Autodesk Fusion 360 part; units mm, degrees
(part 13 of 25)
  line L970 (11.6574, 39.243) -> (5.5534, 39.243)
  arc A2948 (37.4455, 40.2654) -> (37.4455, 40.5829) centre (37.4455, 40.4241) ccw
  line L971 (12.0775, 39.069) -> (11.6574, 39.243)
  line L972 (15.3804, 34.8514) -> (15.113, 35.1188)
  arc A2949 (35.1854, 41.2945) -> (35.5029, 41.2945) centre (35.3441, 41.2945) ccw
  line L973 (15.6337, 33.5781) -> (15.6337, 34.2399)
  line L974 (27.2855, 40.4241) -> (28.1559, 41.2945)
  arc A2950 (38.4746, 42.5255) -> (38.1571, 42.5255) centre (38.3158, 42.5255) ccw
  arc A2951 (5.4412, 39.1307) -> (5.6657, 39.3553) centre (5.5535, 39.243) ccw
  line L975 (26.5671, 40.4241) -> (27.2855, 40.4241)
  line L976 (35.3441, 41.2945) -> (36.2145, 40.4241)
  arc A2952 (14.9663, 35.7266) -> (15.2597, 35.8481) centre (15.113, 35.7874) ccw
  line L977 (36.2145, 40.4241) -> (37.4455, 40.4241)
  arc A2953 (12.1897, 39.1812) -> (11.9652, 38.9567) centre (12.0775, 39.069) ccw
  arc A2954 (38.2036, 42.4132) -> (38.4282, 42.6377) centre (38.3159, 42.5255) ccw
  arc A2955 (12.0167, 38.9223) -> (12.1382, 39.2157) centre (12.0775, 39.069) ccw
  arc A2956 (26.5671, 40.5829) -> (26.5671, 40.2654) centre (26.5671, 40.4241) ccw
  arc A2957 (36.3268, 43.2836) -> (36.1023, 43.5082) centre (36.2145, 43.3959) ccw
  arc A2958 (36.2145, 40.5829) -> (36.2145, 40.2654) centre (36.2145, 40.4241) ccw
  arc A2959 (15.2253, 35.2311) -> (15.0007, 35.0066) centre (15.113, 35.1189) ccw
  line L978 (15.6337, 34.2399) -> (15.3804, 34.8514)
  arc A2960 (15.2682, 34.7392) -> (15.4927, 34.9637) centre (15.3805, 34.8514) ccw
  arc A2961 (37.5577, 43.5082) -> (37.3332, 43.2836) centre (37.4455, 43.3959) ccw
  arc A2962 (4.8214, 43.6691) -> (5.1147, 43.5476) centre (4.968, 43.6084) ccw
  arc A2963 (14.9542, 35.1188) -> (15.2717, 35.1188) centre (15.113, 35.1188) ccw
  line L979 (5.1943, 44.7456) -> (4.9681, 45.2917)
  line L980 (0.9017, 44.1544) -> (1.1279, 43.6083)
  arc A2964 (4.4378, 43.3026) -> (4.6623, 43.0781) centre (4.55, 43.1903) ccw
  arc A2965 (0.9812, 43.5476) -> (1.2746, 43.6691) centre (1.1279, 43.6084) ccw
  line L981 (5.1943, 42.2056) -> (4.9681, 42.7517)
  arc A2966 (1.0157, 45.4039) -> (1.2402, 45.1794) centre (1.128, 45.2917) ccw
  arc A2967 (0.755, 44.8063) -> (1.0484, 44.6848) centre (0.9017, 44.7456) ccw
  arc A2968 (4.2037, 40.6787) -> (4.3252, 40.3853) centre (4.2645, 40.532) ccw
  arc A2969 (5.341, 41.5537) -> (5.0476, 41.6752) centre (5.1943, 41.6145) ccw
  line L982 (4.9681, 42.7517) -> (4.5501, 43.1697)
  line L983 (1.5459, 45.7097) -> (1.1279, 45.2917)
  line L984 (1.5459, 43.1903) -> (1.5708, 43.18)
  arc A2970 (1.6582, 45.5974) -> (1.4336, 45.8219) centre (1.5459, 45.7097) ccw
  arc A2971 (4.0647, 46.0826) -> (3.9432, 45.7892) centre (4.004, 45.9359) ccw
  line L985 (4.9681, 45.2917) -> (4.5501, 45.7097)
  arc A2972 (1.2402, 43.7206) -> (1.0157, 43.496) centre (1.1279, 43.6083) ccw
  arc A2973 (0.7429, 44.1544) -> (1.0605, 44.1544) centre (0.9017, 44.1544) ccw
  arc A2974 (5.0803, 40.956) -> (4.8558, 41.1806) centre (4.9681, 41.0683) ccw
  line L986 (4.5501, 43.1903) -> (4.9681, 43.6083)
  line L987 (1.1279, 43.6083) -> (1.5459, 43.1903)
  line L988 (5.1943, 41.6144) -> (5.1943, 42.2056)
  arc A2975 (5.0355, 41.6144) -> (5.353, 41.6144) centre (5.1943, 41.6144) ccw
  arc A2976 (4.6108, 43.0436) -> (4.4894, 43.337) centre (4.5501, 43.1903) ccw
  line L989 (2.092, 45.9359) -> (1.5459, 45.7097)
  arc A2977 (5.341, 44.0937) -> (5.0476, 44.2152) centre (5.1943, 44.1544) ccw
  arc A2978 (4.4893, 45.563) -> (4.6108, 45.8563) centre (4.5501, 45.7097) ccw
  line L990 (4.5501, 43.1697) -> (4.5252, 43.18)
  arc A2979 (2.092, 46.0946) -> (2.092, 45.7771) centre (2.092, 45.9359) ccw
  line L991 (0.9017, 44.7456) -> (0.9017, 44.1544)
  line L992 (1.1279, 45.2917) -> (0.9017, 44.7456)
  arc A2980 (5.0355, 44.1544) -> (5.353, 44.1544) centre (5.1943, 44.1544) ccw
  arc A2981 (4.8558, 45.1794) -> (5.0803, 45.4039) centre (4.9681, 45.2917) ccw
  arc A2982 (4.4644, 43.3267) -> (4.5859, 43.0333) centre (4.5251, 43.18) ccw
  arc A2983 (1.4336, 43.0781) -> (1.6582, 43.3026) centre (1.5459, 43.1904) ccw
  arc A2984 (4.4893, 43.023) -> (4.6108, 43.3163) centre (4.55, 43.1696) ccw
  arc A2985 (1.0605, 44.7456) -> (0.7429, 44.7456) centre (0.9017, 44.7456) ccw
  line L993 (4.5501, 45.7097) -> (4.004, 45.9359)
  arc A2986 (5.353, 42.2056) -> (5.0355, 42.2056) centre (5.1943, 42.2056) ccw
  arc A2987 (1.0484, 44.2152) -> (0.755, 44.0937) centre (0.9017, 44.1544) ccw
  line L994 (4.9681, 41.0683) -> (5.1943, 41.6144)
  arc A2988 (5.1147, 42.8124) -> (4.8214, 42.6909) centre (4.9681, 42.7516) ccw
  arc A2989 (4.8558, 42.6394) -> (5.0803, 42.8639) centre (4.968, 42.7517) ccw
  line L995 (4.5252, 43.18) -> (4.5501, 43.1903)
  arc A2990 (5.0476, 44.6848) -> (5.341, 44.8063) centre (5.1943, 44.7456) ccw
  arc A2991 (4.5859, 43.3267) -> (4.4644, 43.0333) centre (4.5251, 43.18) ccw
  arc A2992 (5.1147, 45.3524) -> (4.8214, 45.2309) centre (4.968, 45.2916) ccw
  arc A2993 (2.1528, 45.7892) -> (2.0313, 46.0826) centre (2.0921, 45.9359) ccw
  arc A2994 (5.353, 44.7456) -> (5.0355, 44.7456) centre (5.1943, 44.7456) ccw
  arc A2995 (4.6108, 40.5036) -> (4.4893, 40.797) centre (4.5501, 40.6503) ccw
  arc A2996 (4.6623, 45.8219) -> (4.4378, 45.5974) centre (4.5501, 45.7097) ccw
  arc A2997 (5.0803, 43.496) -> (4.8558, 43.7206) centre (4.968, 43.6083) ccw
  arc A2998 (5.0476, 42.1448) -> (5.341, 42.2663) centre (5.1943, 42.2056) ccw
  line L996 (5.1943, 44.1544) -> (5.1943, 44.7456)
  arc A2999 (4.8214, 41.1291) -> (5.1147, 41.0076) centre (4.9681, 41.0684) ccw
  line L997 (4.2644, 40.532) -> (4.5501, 40.6503)
  line L998 (4.5501, 40.6503) -> (4.9681, 41.0683)
  arc A3000 (4.004, 45.7771) -> (4.004, 46.0946) centre (4.004, 45.9359) ccw
  arc A3001 (4.6623, 43.2819) -> (4.4378, 43.0574) centre (4.55, 43.1696) ccw
  arc A3002 (1.4852, 45.8563) -> (1.6067, 45.563) centre (1.5459, 45.7097) ccw
  arc A3003 (1.2746, 45.2309) -> (0.9812, 45.3524) centre (1.1279, 45.2917) ccw
  line L999 (4.004, 45.9359) -> (2.092, 45.9359)
  line L1000 (4.9681, 43.6083) -> (5.1943, 44.1544)
  line L1001 (0.9017, 41.6144) -> (1.1279, 41.0683)
  arc A3004 (1.0605, 42.2056) -> (0.7429, 42.2056) centre (0.9017, 42.2056) ccw
  line L1002 (10.9566, 36.957) -> (12.8109, 35.1027)
  arc A3005 (1.9323, 39.4238) -> (2.2257, 39.5453) centre (2.079, 39.4845) ccw
  line L1003 (1.1279, 41.0683) -> (1.5459, 40.6503)
  arc A3006 (1.4851, 43.3163) -> (1.6067, 43.023) centre (1.5459, 43.1696) ccw
  arc A3007 (2.0638, 40.5016) -> (1.7463, 40.5016) centre (1.9051, 40.5016) ccw
  line L1004 (12.8109, 35.1027) -> (12.5596, 34.8514)
  arc A3008 (0.755, 42.2663) -> (1.0484, 42.1448) centre (0.9017, 42.2056) ccw
  arc A3009 (12.4473, 34.9637) -> (12.6718, 34.7392) centre (12.5595, 34.8514) ccw
  arc A3010 (1.6066, 43.337) -> (1.4852, 43.0436) centre (1.5459, 43.1903) ccw
  arc A3011 (4.2233, 37.5648) -> (3.9988, 37.3403) centre (4.111, 37.4526) ccw
  arc A3012 (1.6316, 43.0333) -> (1.5101, 43.3267) centre (1.5708, 43.18) ccw
  arc A3013 (1.6582, 43.0574) -> (1.4336, 43.2819) centre (1.5459, 43.1696) ccw
  line L1005 (4.111, 37.4525) -> (4.4325, 37.131)
  line L1006 (1.905, 39.9046) -> (2.079, 39.4845)
  arc A3014 (1.5101, 43.0333) -> (1.6316, 43.3267) centre (1.5709, 43.18) ccw
  arc A3015 (12.465, 34.2399) -> (12.1476, 34.2399) centre (12.3063, 34.2399) ccw
  arc A3016 (4.7919, 36.8103) -> (4.9134, 37.1037) centre (4.8527, 36.957) ccw
  arc A3017 (4.3203, 37.0188) -> (4.5448, 37.2433) centre (4.4325, 37.1311) ccw
  arc A3018 (1.2402, 41.1806) -> (1.0157, 40.956) centre (1.128, 41.0683) ccw
  arc A3019 (4.4933, 37.2777) -> (4.3718, 36.9843) centre (4.4326, 37.131) ccw
  arc A3020 (1.0157, 42.8639) -> (1.2402, 42.6394) centre (1.128, 42.7517) ccw
  line L1007 (1.5708, 43.18) -> (1.5459, 43.1697)
  arc A3021 (1.0484, 41.6752) -> (0.755, 41.5537) centre (0.9017, 41.6145) ccw
  line L1008 (4.8526, 36.957) -> (10.9566, 36.957)
  line L1009 (1.905, 40.5016) -> (1.905, 39.9046)
  arc A3022 (11.0688, 37.0693) -> (10.8443, 36.8447) centre (10.9566, 36.957) ccw
  arc A3023 (4.4378, 40.7626) -> (4.6623, 40.5381) centre (4.55, 40.6504) ccw
  arc A3024 (1.8442, 40.3549) -> (1.9658, 40.6482) centre (1.905, 40.5016) ccw
  arc A3025 (1.2746, 42.6909) -> (0.9812, 42.8124) centre (1.1279, 42.7516) ccw
  arc A3026 (2.0517, 39.9654) -> (1.7583, 39.8439) centre (1.905, 39.9047) ccw
  arc A3027 (12.1596, 34.3007) -> (12.453, 34.1792) centre (12.3063, 34.24) ccw
  line L1010 (1.5459, 40.6503) -> (1.905, 40.5016)
  arc A3028 (1.4336, 40.5381) -> (1.6582, 40.7626) centre (1.5459, 40.6504) ccw
  arc A3029 (12.9231, 34.9904) -> (12.6986, 35.2149) centre (12.8109, 35.1027) ccw
  line L1011 (0.9017, 42.2056) -> (0.9017, 41.6144)
  line L1012 (12.5596, 34.8514) -> (12.3063, 34.2399)
  line L1013 (1.5459, 43.1697) -> (1.1279, 42.7517)
  line L1014 (2.079, 39.4845) -> (4.111, 37.4525)
  arc A3030 (4.8526, 37.1157) -> (4.8526, 36.7983) centre (4.8526, 36.957) ccw
  line L1015 (4.4325, 37.131) -> (4.8526, 36.957)
  arc A3031 (0.9812, 41.0076) -> (1.2746, 41.1291) centre (1.1279, 41.0684) ccw
  arc A3032 (0.7429, 41.6144) -> (1.0605, 41.6144) centre (0.9017, 41.6144) ccw
  arc A3033 (3.9988, 37.3403) -> (4.2233, 37.5648) centre (4.111, 37.4526) ccw
  arc A3034 (10.9566, 36.7983) -> (10.9566, 37.1157) centre (10.9566, 36.957) ccw
  arc A3035 (1.7463, 39.9046) -> (2.0638, 39.9046) centre (1.9051, 39.9046) ccw
  arc A3036 (1.6067, 40.797) -> (1.4852, 40.5036) centre (1.5459, 40.6503) ccw
  line L1016 (1.1279, 42.7517) -> (0.9017, 42.2056)
  arc A3037 (15.2337, 33.0273) -> (15.5271, 32.9058) centre (15.3804, 32.9666) ccw
  line L1017 (15.3797, 3.81) -> (15.3797, 4.3939)
  arc A3038 (15.7459, 5.5486) -> (15.5214, 5.7731) centre (15.6337, 5.6609) ccw
  arc A3039 (13.8112, 2.4003) -> (14.1287, 2.4003) centre (13.97, 2.4003) ccw
  arc A3040 (12.6986, 34.9904) -> (12.9231, 35.2149) centre (12.8109, 35.1027) ccw
  line L1018 (15.3804, 32.9666) -> (15.6337, 33.5781)
  arc A3041 (13.0883, 32.6452) -> (12.9668, 32.3519) centre (13.0275, 32.4986) ccw
  arc A3042 (13.97, 3.9688) -> (13.97, 3.6513) centre (13.97, 3.81) ccw
  arc A3043 (13.97, 3.9687) -> (13.97, 3.6512) centre (13.97, 3.81) ccw
  line L1019 (14.5539, 2.4003) -> (15.3797, 3.2261)
  arc A3044 (15.3797, 3.6513) -> (15.3797, 3.9688) centre (15.3797, 3.81) ccw
  arc A3045 (15.7804, 33.5173) -> (15.487, 33.6388) centre (15.6337, 33.578) ccw
  arc A3046 (13.6391, 32.404) -> (13.6391, 32.0866) centre (13.6391, 32.2453) ccw
  line L1020 (13.97, 2.4003) -> (13.97, 3.81)
  arc A3047 (12.6718, 33.0788) -> (12.4473, 32.8543) centre (12.5596, 32.9666) ccw
  arc A3048 (15.2209, 3.81) -> (15.5384, 3.81) centre (15.3796, 3.81) ccw
  line L1021 (13.0276, 32.4986) -> (13.6391, 32.2453)
  line L1022 (15.3797, 4.3939) -> (14.8732, 4.9004)
  arc A3049 (15.2674, 4.2817) -> (15.492, 4.5062) centre (15.3797, 4.394) ccw
  arc A3050 (13.97, 3.9687) -> (13.97, 3.6512) centre (13.97, 3.81) ccw
  arc A3051 (15.5384, 4.3939) -> (15.2209, 4.3939) centre (15.3796, 4.3939) ccw
  arc A3052 (2.1913, 39.5968) -> (1.9668, 39.3723) centre (2.0791, 39.4846) ccw
  line L1023 (13.97, 3.81) -> (15.3797, 3.81)
  line L1024 (14.8732, 4.9004) -> (15.6337, 5.6609)
  arc A3053 (14.9732, 32.3519) -> (14.8517, 32.6452) centre (14.9124, 32.4986) ccw
  arc A3054 (12.4129, 32.9058) -> (12.7062, 33.0273) centre (12.5596, 32.9666) ccw
  line L1025 (15.6337, 5.6609) -> (15.6337, 7.0391)
  arc A3055 (13.97, 2.2415) -> (13.97, 2.559) centre (13.97, 2.4003) ccw
  arc A3056 (15.5384, 3.81) -> (15.2209, 3.81) centre (15.3796, 3.81) ccw
  arc A3057 (12.453, 33.6388) -> (12.1596, 33.5173) centre (12.3063, 33.578) ccw
  line L1026 (12.5596, 32.9666) -> (13.0276, 32.4986)
  arc A3058 (13.97, 3.6512) -> (13.97, 3.9687) centre (13.97, 3.81) ccw
  arc A3059 (12.9153, 32.3863) -> (13.1398, 32.6108) centre (13.0275, 32.4986) ccw
  line L1027 (15.3797, 3.2261) -> (15.3797, 3.81)
  line L1028 (13.3861, 2.4003) -> (13.97, 2.4003)
  arc A3060 (10.7132, 8.4483) -> (10.4887, 8.2238) centre (10.601, 8.3361) ccw
  line L1029 (6.2035, 16.2179) -> (5.6955, 16.7259)
  arc A3061 (10.5988, 8.7562) -> (10.3054, 8.6347) centre (10.4521, 8.6955) ccw
  line L1030 (12.3063, 6.6307) -> (12.3063, 5.6609)
  arc A3062 (11.8717, 12.1468) -> (12.0962, 12.3713) centre (11.984, 12.2591) ccw
  arc A3063 (14.1288, 3.81) -> (13.8113, 3.81) centre (13.9701, 3.81) ccw
  line L1031 (14.3009, 32.2453) -> (14.9124, 32.4986)
  arc A3064 (15.2209, 3.2261) -> (15.5384, 3.2261) centre (15.3796, 3.2261) ccw
  line L1032 (4.4645, 13.7541) -> (5.6955, 13.7541)
  line L1033 (12.4079, 9.2951) -> (12.4079, 11.6245)
  arc A3065 (14.8002, 32.6108) -> (15.0247, 32.3863) centre (14.9125, 32.4986) ccw
  line L1034 (7.2149, 14.2621) -> (10.4521, 11.0249)
  arc A3066 (13.97, 2.5591) -> (13.97, 2.2416) centre (13.97, 2.4004) ccw
  arc A3067 (14.761, 5.0126) -> (14.9855, 4.7881) centre (14.8733, 4.9003) ccw
  arc A3068 (14.2402, 32.392) -> (14.3617, 32.0986) centre (14.301, 32.2453) ccw
  line L1035 (13.97, 3.81) -> (13.97, 2.4003)
  arc A3069 (13.3861, 2.559) -> (13.3861, 2.2416) centre (13.3861, 2.4003) ccw
  line L1036 (15.3797, 3.81) -> (13.97, 3.81)
  arc A3070 (13.5783, 32.0986) -> (13.6998, 32.392) centre (13.639, 32.2453) ccw
  arc A3071 (14.1288, 3.81) -> (13.8113, 3.81) centre (13.9701, 3.81) ccw
  arc A3072 (15.4927, 32.8543) -> (15.2682, 33.0788) centre (15.3804, 32.9666) ccw
  arc A3073 (4.4645, 13.9129) -> (4.4645, 13.5954) centre (4.4645, 13.7542) ccw
  arc A3074 (12.0962, 12.3713) -> (11.8717, 12.1468) centre (11.984, 12.2591) ccw
  arc A3075 (15.4749, 5.6609) -> (15.7924, 5.6609) centre (15.6337, 5.6609) ccw
  arc A3076 (8.2862, 16.1813) -> (8.0617, 15.9568) centre (8.1739, 16.0691) ccw
  arc A3077 (7.3272, 14.3744) -> (7.1027, 14.1498) centre (7.2149, 14.2621) ccw
  arc A3078 (15.492, 3.1138) -> (15.2674, 3.3383) centre (15.3797, 3.2261) ccw
  line L1037 (13.97, 2.4003) -> (14.5539, 2.4003)
  arc A3079 (14.9855, 5.0126) -> (14.761, 4.7881) centre (14.8733, 4.9003) ccw
  arc A3080 (14.1287, 3.81) -> (13.8112, 3.81) centre (13.97, 3.81) ccw
  line L1038 (14.9124, 32.4986) -> (15.3804, 32.9666)
  arc A3081 (7.8145, 16.0591) -> (7.8145, 16.3766) centre (7.8145, 16.2179) ccw
  arc A3082 (12.5666, 11.6245) -> (12.2491, 11.6245) centre (12.4078, 11.6245) ccw
  line L1039 (15.6337, 7.0391) -> (14.6591, 8.0137)
  line L1040 (12.4079, 11.6245) -> (12.259, 11.9839)
  arc A3083 (3.7529, 15.8555) -> (3.4354, 15.8555) centre (3.5941, 15.8555) ccw
  line L1041 (10.4521, 11.0249) -> (10.4521, 8.6955)
  arc A3084 (10.6108, 11.0249) -> (10.2934, 11.0249) centre (10.4521, 11.0249) ccw
  arc A3085 (10.4543, 8.2753) -> (10.7476, 8.3968) centre (10.601, 8.3361) ccw
  arc A3086 (72.6868, 22.0663) -> (72.6868, 22.3838) centre (72.6868, 22.2251) ccw
  arc A3087 (5.6955, 13.5954) -> (5.6955, 13.9129) centre (5.6955, 13.7542) ccw
  arc A3088 (14.3009, 32.0866) -> (14.3009, 32.404) centre (14.3009, 32.2453) ccw
  arc A3089 (56.8579, 22.3838) -> (56.8579, 22.0663) centre (56.8579, 22.2251) ccw
  arc A3090 (15.3797, 3.6512) -> (15.3797, 3.9687) centre (15.3797, 3.81) ccw
  arc A3091 (7.2149, 14.1034) -> (7.2149, 14.4208) centre (7.2149, 14.2621) ccw
  arc A3092 (14.5539, 2.2416) -> (14.5539, 2.5591) centre (14.5539, 2.4004) ccw
  arc A3093 (4.4645, 16.8846) -> (4.4645, 16.5671) centre (4.4645, 16.7259) ccw
  arc A3094 (15.7924, 7.0391) -> (15.4749, 7.0391) centre (15.6337, 7.0391) ccw
  arc A3095 (14.4417, 2.5126) -> (14.6662, 2.288) centre (14.554, 2.4003) ccw
  arc A3096 (13.8113, 3.81) -> (14.1288, 3.81) centre (13.9701, 3.81) ccw
  arc A3097 (13.8113, 2.4003) -> (14.1288, 2.4003) centre (13.9701, 2.4003) ccw
  line L1042 (13.6391, 32.2453) -> (14.3009, 32.2453)
  arc A3098 (6.2035, 16.3766) -> (6.2035, 16.0591) centre (6.2035, 16.2179) ccw
  line L1043 (3.5941, 14.6245) -> (4.4645, 13.7541)
  arc A3099 (12.1476, 5.6609) -> (12.465, 5.6609) centre (12.3063, 5.6609) ccw
  line L1044 (10.4521, 8.6955) -> (10.601, 8.3361)
  arc A3100 (44.8038, 14.6194) -> (44.5105, 14.7409) centre (44.6572, 14.6802) ccw
  arc A3101 (44.6251, 14.2194) -> (44.3076, 14.2194) centre (44.4664, 14.2194) ccw
  line L1045 (13.6893, 8.0137) -> (12.4079, 9.2951)
  line L1046 (12.5603, 3.2261) -> (13.3861, 2.4003)
  arc A3102 (12.2612, 11.5638) -> (12.5546, 11.6853) centre (12.4079, 11.6246) ccw
  line L1047 (13.0668, 4.9004) -> (12.5603, 4.3939)
  arc A3103 (45.5314, 15.077) -> (45.4099, 15.3704) centre (45.4706, 15.2237) ccw
  arc A3104 (3.4354, 14.6245) -> (3.7529, 14.6245) centre (3.5941, 14.6245) ccw
  line L1048 (44.4663, 13.7206) -> (44.6572, 13.2598)
  arc A3105 (13.6893, 8.1724) -> (13.6893, 7.8549) centre (13.6893, 8.0137) ccw
  arc A3106 (14.7714, 8.126) -> (14.5469, 7.9014) centre (14.6592, 8.0137) ccw
  arc A3107 (12.2491, 9.2951) -> (12.5666, 9.2951) centre (12.4078, 9.2951) ccw
  arc A3108 (6.2035, 14.4208) -> (6.2035, 14.1034) centre (6.2035, 14.2621) ccw
  line L1049 (3.5941, 15.8555) -> (3.5941, 14.6245)
  arc A3109 (8.1132, 15.9224) -> (8.2347, 16.2157) centre (8.1739, 16.0691) ccw
  arc A3110 (6.0912, 16.1056) -> (6.3157, 16.3302) centre (6.2035, 16.2179) ccw
  line L1050 (7.8145, 16.2179) -> (6.2035, 16.2179)
  arc A3111 (4.3523, 13.6418) -> (4.5768, 13.8664) centre (4.4646, 13.7541) ccw
  arc A3112 (12.5202, 9.4073) -> (12.2956, 9.1828) centre (12.4079, 9.2951) ccw
  arc A3113 (12.1468, 11.8717) -> (12.3713, 12.0962) centre (12.2591, 11.984) ccw
  arc A3114 (14.6591, 7.8549) -> (14.6591, 8.1724) centre (14.6591, 8.0137) ccw
  arc A3115 (7.8753, 16.3646) -> (7.7538, 16.0712) centre (7.8146, 16.2179) ccw
  arc A3116 (4.5768, 16.6136) -> (4.3523, 16.8382) centre (4.4645, 16.7259) ccw
  arc A3117 (10.3398, 10.9127) -> (10.5644, 11.1372) centre (10.4521, 11.025) ccw
  arc A3118 (5.6955, 16.5671) -> (5.6955, 16.8846) centre (5.6955, 16.7259) ccw
  line L1051 (14.6591, 8.0137) -> (13.6893, 8.0137)
  arc A3119 (5.5832, 13.8664) -> (5.8077, 13.6418) centre (5.6954, 13.7541) ccw
  arc A3120 (44.3076, 13.7206) -> (44.6251, 13.7206) centre (44.4664, 13.7206) ccw
  arc A3121 (44.3196, 14.2801) -> (44.613, 14.1586) centre (44.4663, 14.2193) ccw
  line L1052 (5.6955, 16.7259) -> (4.4645, 16.7259)
  arc A3122 (3.4818, 15.9677) -> (3.7064, 15.7432) centre (3.5941, 15.8554) ccw
  line L1053 (12.259, 11.9839) -> (11.9839, 12.259)
  arc A3123 (3.7064, 14.7368) -> (3.4818, 14.5123) centre (3.5941, 14.6246) ccw
  line L1054 (45.4706, 15.2237) -> (45.0098, 15.0328)
  arc A3124 (12.4057, 12.0447) -> (12.1124, 11.9232) centre (12.2591, 11.984) ccw
  arc A3125 (12.4016, 3.81) -> (12.719, 3.81) centre (12.5603, 3.81) ccw
  arc A3126 (14.1287, 3.81) -> (13.8112, 3.81) centre (13.97, 3.81) ccw
  line L1055 (12.5603, 3.81) -> (13.97, 3.81)
  line L1056 (5.6955, 13.7541) -> (6.2035, 14.2621)
  arc A3127 (5.8077, 16.8382) -> (5.5832, 16.6136) centre (5.6954, 16.7259) ccw
  line L1057 (12.3063, 5.6609) -> (13.0668, 4.9004)
  line L1058 (12.5603, 4.3939) -> (12.5603, 3.81)
  line L1059 (6.2035, 14.2621) -> (7.2149, 14.2621)
  line L1060 (8.1739, 16.069) -> (7.8145, 16.2179)
  arc A3128 (6.3157, 14.1498) -> (6.0912, 14.3744) centre (6.2035, 14.2621) ccw
  line L1061 (44.6572, 13.2598) -> (44.7421, 13.1749)
  line L1062 (10.601, 8.3361) -> (12.3063, 6.6307)
  arc A3129 (44.5105, 13.1991) -> (44.8038, 13.3206) centre (44.6572, 13.2599) ccw
  arc A3130 (10.2934, 8.6955) -> (10.6108, 8.6955) centre (10.4521, 8.6955) ccw
  line L1063 (11.9839, 12.259) -> (8.1739, 16.069)
  arc A3131 (12.4016, 3.2261) -> (12.719, 3.2261) centre (12.5603, 3.2261) ccw
  line L1064 (4.4645, 16.7259) -> (3.5941, 15.8555)
  arc A3132 (15.5214, 6.9269) -> (15.746, 7.1514) centre (15.6337, 7.0391) ccw
  arc A3133 (13.577, 7.9014) -> (13.8015, 8.1259) centre (13.6893, 8.0137) ccw
  arc A3134 (12.5603, 3.9688) -> (12.5603, 3.6513) centre (12.5603, 3.81) ccw
  arc A3135 (46.8149, 13.7206) -> (47.1324, 13.7206) centre (46.9737, 13.7206) ccw
  arc A3136 (12.194, 6.5185) -> (12.4186, 6.743) centre (12.3063, 6.6308) ccw
  arc A3137 (44.7694, 13.3721) -> (44.5449, 13.1476) centre (44.6571, 13.2599) ccw
  arc A3138 (12.465, 6.6307) -> (12.1476, 6.6307) centre (12.3063, 6.6307) ccw
  arc A3139 (44.6298, 13.0626) -> (44.8544, 13.2872) centre (44.7421, 13.1749) ccw
  line L1065 (44.7421, 13.1749) -> (44.7421, 7.8557)
  arc A3140 (44.8028, 7.709) -> (44.6814, 8.0024) centre (44.7421, 7.8557) ccw
  arc A3141 (44.9008, 13.1749) -> (44.5834, 13.1749) centre (44.7421, 13.1749) ccw
  arc A3142 (45.9694, 15.0649) -> (45.9694, 15.3824) centre (45.9694, 15.2236) ccw
  arc A3143 (13.2738, 2.288) -> (13.4983, 2.5126) centre (13.3861, 2.4003) ccw
  arc A3144 (40.0108, 7.9016) -> (40.1089, 7.5996) centre (40.0599, 7.7506) ccw
  arc A3145 (46.5424, 15.1451) -> (46.3179, 14.9206) centre (46.4301, 15.0329) ccw
  line L1066 (44.6572, 14.6802) -> (44.4663, 14.2194)
  arc A3146 (44.6593, 7.9932) -> (44.7808, 7.6999) centre (44.7201, 7.8466) ccw
  arc A3147 (43.5919, 8.262) -> (43.4704, 7.9686) centre (43.5312, 8.1153) ccw
  arc A3148 (44.1192, 7.6999) -> (44.2407, 7.9932) centre (44.1799, 7.8466) ccw
  arc A3149 (13.179, 4.7881) -> (12.9545, 5.0126) centre (13.0668, 4.9003) ccw
  arc A3150 (43.5311, 7.9565) -> (43.5311, 8.274) centre (43.5311, 8.1152) ccw
  arc A3151 (46.6706, 14.5679) -> (46.8951, 14.7924) centre (46.7829, 14.6801) ccw
  line L1067 (46.4302, 15.0328) -> (45.9694, 15.2237)
  arc A3152 (46.0301, 15.3704) -> (45.9086, 15.077) centre (45.9694, 15.2237) ccw
  line L1068 (45.9694, 15.2237) -> (45.4706, 15.2237)
  arc A3153 (46.9295, 14.7409) -> (46.6362, 14.6194) centre (46.7828, 14.6801) ccw
  arc A3154 (12.719, 4.3939) -> (12.4016, 4.3939) centre (12.5603, 4.3939) ccw
  line L1069 (12.5603, 3.81) -> (12.5603, 3.2261)
  arc A3155 (45.4706, 15.3824) -> (45.4706, 15.0649) centre (45.4706, 15.2236) ccw
  arc A3156 (47.1324, 14.2194) -> (46.8149, 14.2194) centre (46.9737, 14.2194) ccw
  arc A3157 (44.5834, 7.8557) -> (44.9008, 7.8557) centre (44.7421, 7.8557) ccw
  arc A3158 (12.6726, 3.3383) -> (12.448, 3.1138) centre (12.5603, 3.2261) ccw
  arc A3159 (13.97, 3.6513) -> (13.97, 3.9688) centre (13.97, 3.81) ccw
  line L1070 (46.9737, 14.2194) -> (46.7828, 14.6802)
  arc A3160 (46.3694, 14.8862) -> (46.4909, 15.1795) centre (46.4301, 15.0328) ccw
  arc A3161 (44.5449, 14.7924) -> (44.7694, 14.5679) centre (44.6571, 14.6802) ccw
  line L1071 (44.72, 7.8465) -> (44.45, 7.5765)
  line L1072 (44.7421, 7.8557) -> (44.72, 7.8465)
  line L1073 (44.4663, 14.2194) -> (44.4663, 13.7206)
  line L1074 (45.0098, 15.0328) -> (44.6572, 14.6802)
  line L1075 (39.6555, 7.5028) -> (39.4872, 7.3345)
  line L1076 (46.7828, 14.6802) -> (46.4302, 15.0328)
  arc A3162 (44.613, 13.7814) -> (44.3196, 13.6599) centre (44.4663, 13.7206) ccw
  arc A3163 (13.97, 3.6512) -> (13.97, 3.9687) centre (13.97, 3.81) ccw
  arc A3164 (12.4186, 5.7731) -> (12.194, 5.5486) centre (12.3063, 5.6609) ccw
  line L1077 (40.2861, 7.8241) -> (40.0599, 7.7506)
  line L1078 (46.9737, 13.7206) -> (46.9737, 14.2194)
  arc A3165 (41.6181, 7.5092) -> (41.8426, 7.2846) centre (41.7303, 7.3969) ccw
  arc A3166 (45.1221, 14.9206) -> (44.8976, 15.1451) centre (45.0099, 15.0328) ccw
  arc A3167 (39.375, 7.4468) -> (39.5995, 7.2223) centre (39.4873, 7.3346) ccw
  arc A3168 (12.719, 3.81) -> (12.4016, 3.81) centre (12.5603, 3.81) ccw
  arc A3169 (13.8112, 3.81) -> (14.1287, 3.81) centre (13.97, 3.81) ccw
  arc A3170 (40.9691, 7.6673) -> (41.0187, 7.9809) centre (40.9939, 7.8241) ccw
  line L1079 (43.5311, 8.1153) -> (42.8289, 8.1153)
  arc A3171 (42.8896, 7.9686) -> (42.7681, 8.262) centre (42.8289, 8.1153) ccw
  line L1080 (13.97, 3.81) -> (12.5603, 3.81)
  arc A3172 (44.9491, 15.1795) -> (45.0706, 14.8862) centre (45.0099, 15.0328) ccw
  arc A3173 (42.2923, 7.7343) -> (42.0678, 7.9588) centre (42.18, 7.8466) ccw
  arc A3174 (12.9545, 4.7881) -> (13.179, 5.0126) centre (13.0668, 4.9003) ccw
  arc A3175 (40.64, 8.02) -> (40.64, 7.7025) centre (40.64, 7.8613) ccw
  line L1081 (41.2201, 7.7506) -> (40.9939, 7.8241)
  arc A3176 (12.448, 4.5062) -> (12.6726, 4.2817) centre (12.5603, 4.394) ccw
  line L1082 (40.9939, 7.8241) -> (40.7589, 7.8613)
  arc A3177 (46.827, 14.1586) -> (47.1204, 14.2801) centre (46.9737, 14.2194) ccw
  arc A3178 (41.7368, 7.615) -> (41.5123, 7.3905) centre (41.6246, 7.5027) ccw
  arc A3179 (12.5603, 3.9687) -> (12.5603, 3.6512) centre (12.5603, 3.81) ccw
  arc A3180 (39.7677, 7.3905) -> (39.5432, 7.615) centre (39.6555, 7.5028) ccw
  line L1083 (42.8289, 8.1153) -> (42.18, 7.8465)
  arc A3181 (40.7987, 7.8613) -> (40.4812, 7.8613) centre (40.6399, 7.8613) ccw
  arc A3182 (41.5312, 7.3743) -> (41.7179, 7.6312) centre (41.6246, 7.5027) ccw
  arc A3183 (41.36, 7.5011) -> (41.5042, 7.784) centre (41.4321, 7.6425) ccw
  arc A3184 (40.7988, 7.8613) -> (40.4813, 7.8613) centre (40.6401, 7.8613) ccw
  arc A3185 (40.64, 6.1913) -> (40.64, 6.5088) centre (40.64, 6.3501) ccw
  arc A3186 (39.2416, 7.2665) -> (39.4984, 7.0799) centre (39.37, 7.1732) ccw
  arc A3187 (34.6723, 7.7343) -> (34.4478, 7.9588) centre (34.5601, 7.8466) ccw
  arc A3188 (41.043, 7.9751) -> (40.9448, 7.6731) centre (40.9939, 7.8241) ccw
  arc A3189 (38.2438, 8.0181) -> (38.1941, 7.7045) centre (38.2189, 7.8613) ccw
  arc A3190 (41.2922, 7.892) -> (41.1481, 7.6091) centre (41.2202, 7.7506) ccw
  arc A3191 (35.2696, 7.9686) -> (35.1481, 8.262) centre (35.2088, 8.1153) ccw
  line L1084 (40.0599, 7.7506) -> (39.8479, 7.6426)
  arc A3192 (42.8289, 8.274) -> (42.8289, 7.9565) centre (42.8289, 8.1152) ccw
  line L1085 (35.9111, 8.1153) -> (35.2089, 8.1153)
  arc A3193 (38.1, 7.7025) -> (38.1, 8.02) centre (38.1, 7.8613) ccw
  arc A3194 (38.9912, 7.3743) -> (39.1779, 7.6312) centre (39.0846, 7.5028) ccw
  line L1086 (37.7461, 7.8241) -> (37.5199, 7.7506)
  arc A3195 (40.5211, 8.02) -> (40.5211, 7.7025) centre (40.5211, 7.8613) ccw
  arc A3196 (37.2358, 7.784) -> (37.38, 7.5011) centre (37.3079, 7.6425) ccw
  line L1087 (41.7304, 7.3969) -> (41.6245, 7.5028)
  arc A3197 (38.2189, 7.7025) -> (38.2189, 8.02) centre (38.2189, 7.8613) ccw
  line L1088 (37.1155, 7.5028) -> (37.0096, 7.3969)
  arc A3198 (41.6181, 7.2846) -> (41.8426, 7.5092) centre (41.7304, 7.3969) ccw
  line L1089 (39.37, 7.1732) -> (39.2528, 7.3345)
  arc A3199 (38.1, 8.02) -> (38.1, 7.7025) centre (38.1, 7.8613) ccw
  arc A3200 (35.2089, 8.274) -> (35.2089, 7.9565) centre (35.2089, 8.1152) ccw
  line L1090 (39.4872, 7.3345) -> (39.37, 7.1732)
  arc A3201 (37.0221, 7.6312) -> (37.2088, 7.3743) centre (37.1155, 7.5028) ccw
  line L1091 (40.64, 7.8613) -> (40.64, 6.35)
  arc A3202 (38.6311, 7.5996) -> (38.7292, 7.9016) centre (38.6802, 7.7506) ccw
  arc A3203 (40.7838, 8.0181) -> (40.7341, 7.7045) centre (40.7589, 7.8613) ccw
  arc A3204 (36.8973, 7.2846) -> (37.1219, 7.5092) centre (37.0096, 7.3969) ccw
  line L1092 (44.45, 7.5765) -> (44.18, 7.8465)
  line L1093 (39.8479, 7.6426) -> (39.6555, 7.5028)
  arc A3205 (40.1319, 7.6091) -> (39.9878, 7.892) centre (40.0599, 7.7506) ccw
  arc A3206 (40.64, 7.7025) -> (40.64, 8.02) centre (40.64, 7.8613) ccw
  arc A3207 (39.6157, 7.2412) -> (39.3588, 7.4279) centre (39.4873, 7.3346) ccw
  arc A3208 (40.7589, 7.7025) -> (40.7589, 8.02) centre (40.7589, 7.8613) ccw
  line L1094 (40.64, 7.8613) -> (40.5211, 7.8613)
  line L1095 (41.4321, 7.6426) -> (41.2201, 7.7506)
  arc A3209 (39.9412, 7.5141) -> (39.7546, 7.771) centre (39.8479, 7.6425) ccw
  arc A3210 (40.4813, 6.35) -> (40.7988, 6.35) centre (40.6401, 6.35) ccw
  arc A3211 (44.3377, 7.4643) -> (44.5623, 7.6888) centre (44.45, 7.5766) ccw
  line L1096 (41.6245, 7.5028) -> (41.4321, 7.6426)
  arc A3212 (44.3377, 7.6888) -> (44.5623, 7.4643) centre (44.45, 7.5766) ccw
  arc A3213 (40.64, 6.5088) -> (40.64, 6.1913) centre (40.64, 6.3501) ccw
  line L1097 (40.7589, 7.8613) -> (40.64, 7.8613)
  line L1098 (37.9811, 7.8613) -> (37.7461, 7.8241)
  line L1099 (40.5211, 7.8613) -> (40.2861, 7.8241)
  arc A3214 (44.8323, 7.7343) -> (44.6078, 7.9588) centre (44.72, 7.8466) ccw
  arc A3215 (41.5254, 7.771) -> (41.3388, 7.5141) centre (41.4321, 7.6426) ccw
  line L1100 (38.1, 6.35) -> (38.1, 7.8613)
  line L1101 (40.64, 6.35) -> (40.64, 7.8613)
  arc A3216 (40.3352, 7.6731) -> (40.237, 7.9751) centre (40.2861, 7.8241) ccw
  arc A3217 (42.1193, 7.9932) -> (42.2408, 7.6999) centre (42.18, 7.8465) ccw
  arc A3218 (41.1711, 7.5996) -> (41.2692, 7.9016) centre (41.2202, 7.7506) ccw
  line L1102 (44.18, 7.8465) -> (43.5311, 8.1153)
  arc A3219 (40.5459, 7.7045) -> (40.4962, 8.0181) centre (40.5211, 7.8613) ccw
  arc A3220 (44.2922, 7.9588) -> (44.0677, 7.7343) centre (44.18, 7.8465) ccw
  arc A3221 (39.7758, 7.784) -> (39.92, 7.5011) centre (39.8479, 7.6426) ccw
  arc A3222 (34.1777, 7.6888) -> (34.4023, 7.4643) centre (34.29, 7.5765) ccw
  arc A3223 (40.2613, 7.9809) -> (40.3109, 7.6673) centre (40.2861, 7.8241) ccw
  line L1103 (37.5199, 7.7506) -> (37.3079, 7.6426)
  arc A3224 (39.5621, 7.6312) -> (39.7488, 7.3743) centre (39.6555, 7.5028) ccw
  line L1104 (34.56, 7.8465) -> (34.29, 7.5765)
  arc A3225 (40.4812, 6.35) -> (40.7987, 6.35) centre (40.6399, 6.35) ccw
  line L1105 (42.18, 7.8465) -> (41.7304, 7.3969)
  arc A3226 (38.9854, 7.771) -> (38.7988, 7.5141) centre (38.8921, 7.6425) ccw
  arc A3227 (34.4993, 7.9932) -> (34.6208, 7.6999) centre (34.5601, 7.8466) ccw
  arc A3228 (37.4708, 7.9016) -> (37.5689, 7.5996) centre (37.5199, 7.7506) ccw
  arc A3229 (36.4992, 7.6999) -> (36.6207, 7.9932) centre (36.5599, 7.8466) ccw
  arc A3230 (38.7522, 7.892) -> (38.6081, 7.6091) centre (38.6802, 7.7505) ccw
  arc A3231 (38.4291, 7.6673) -> (38.4787, 7.9809) centre (38.4539, 7.8241) ccw
  arc A3232 (36.8973, 7.5092) -> (37.1219, 7.2846) centre (37.0096, 7.3969) ccw
  arc A3233 (37.5919, 7.6091) -> (37.4478, 7.892) centre (37.5199, 7.7506) ccw
  arc A3234 (39.1968, 7.615) -> (38.9723, 7.3905) centre (39.0846, 7.5028) ccw
  line L1106 (38.2189, 7.8613) -> (38.1, 7.8613)
  line L1107 (29.21, 15.2835) -> (29.48, 15.0135)
  arc A3235 (37.7213, 7.9809) -> (37.7709, 7.6673) centre (37.7461, 7.8241) ccw
  arc A3236 (29.3678, 14.9012) -> (29.5923, 15.1257) centre (29.4801, 15.0135) ccw
  line L1108 (31.6665, 7.493) -> (30.9534, 7.493)
  line L1109 (38.1, 7.8613) -> (38.1, 6.35)
  arc A3237 (38.503, 7.9751) -> (38.4048, 7.6731) centre (38.4539, 7.8241) ccw
  arc A3238 (35.9719, 8.262) -> (35.8504, 7.9686) centre (35.9112, 8.1153) ccw
  arc A3239 (37.9811, 8.02) -> (37.9811, 7.7025) centre (37.9811, 7.8613) ccw
  line L1110 (26.4, 15.0135) -> (26.67, 15.2835)
  arc A3240 (25.6904, 14.8914) -> (25.8119, 14.598) centre (25.7512, 14.7447) ccw
  arc A3241 (30.0681, 14.598) -> (30.1896, 14.8914) centre (30.1288, 14.7447) ccw
  arc A3242 (37.9413, 6.35) -> (38.2588, 6.35) centre (38.1, 6.35) ccw
  arc A3243 (39.3812, 7.4279) -> (39.1243, 7.2412) centre (39.2527, 7.3346) ccw
  arc A3244 (37.4012, 7.5141) -> (37.2146, 7.771) centre (37.3079, 7.6425) ccw
  line L1111 (30.1289, 14.7447) -> (30.8311, 14.7447)
  arc A3245 (38.1, 6.5088) -> (38.1, 6.1913) centre (38.1, 6.3501) ccw
  arc A3246 (23.8907, 15.2687) -> (24.1153, 15.0442) centre (24.003, 15.1565) ccw
  arc A3247 (24.2423, 15.3957) -> (24.0177, 15.1712) centre (24.13, 15.2835) ccw
  arc A3248 (34.1777, 7.4643) -> (34.4023, 7.6888) centre (34.29, 7.5765) ccw
  line L1112 (38.4539, 7.8241) -> (38.2189, 7.8613)
  arc A3249 (39.1405, 7.2223) -> (39.365, 7.4468) centre (39.2528, 7.3346) ccw
  arc A3250 (26.7823, 15.1712) -> (26.5577, 15.3957) centre (26.67, 15.2835) ccw
  line L1113 (24.13, 15.2835) -> (24.4, 15.0135)
  line L1114 (25.0489, 14.7447) -> (25.7511, 14.7447)
  line L1115 (39.2528, 7.3345) -> (39.0845, 7.5028)
  arc A3251 (38.2588, 7.8613) -> (37.9413, 7.8613) centre (38.1, 7.8613) ccw
  arc A3252 (25.0489, 14.9034) -> (25.0489, 14.586) centre (25.0489, 14.7447) ccw
  arc A3253 (29.3223, 15.1712) -> (29.0977, 15.3957) centre (29.21, 15.2835) ccw
  arc A3254 (26.2877, 15.1257) -> (26.5122, 14.9012) centre (26.4, 15.0135) ccw
  line L1116 (39.0845, 7.5028) -> (38.8921, 7.6426)
  arc A3255 (29.3223, 15.3957) -> (29.0977, 15.1712) centre (29.21, 15.2834) ccw
  arc A3256 (38.2587, 7.8613) -> (37.9412, 7.8613) centre (38.0999, 7.8613) ccw
  line L1117 (25.7511, 14.7447) -> (26.4, 15.0135)
  line L1118 (37.0096, 7.3969) -> (36.56, 7.8465)
  arc A3257 (29.5408, 15.1601) -> (29.4193, 14.8668) centre (29.4801, 15.0135) ccw
  arc A3258 (31.6665, 7.3342) -> (31.6665, 7.6517) centre (31.6665, 7.493) ccw
  arc A3259 (34.1322, 7.9588) -> (33.9077, 7.7343) centre (34.02, 7.8466) ccw
  line L1119 (36.56, 7.8465) -> (35.9111, 8.1153)
  line L1120 (34.29, 7.5765) -> (34.02, 7.8465)
  arc A3260 (38.1, 6.1913) -> (38.1, 6.5088) centre (38.1, 6.3501) ccw
  line L1121 (28.94, 15.0135) -> (29.21, 15.2835)
  arc A3261 (37.7952, 7.6731) -> (37.697, 7.9751) centre (37.7461, 7.8241) ccw
  arc A3262 (37.9412, 6.35) -> (38.2587, 6.35) centre (38.0999, 6.35) ccw
  arc A3263 (35.9111, 7.9565) -> (35.9111, 8.274) centre (35.9111, 8.1152) ccw
  line L1122 (38.1, 7.8613) -> (37.9811, 7.8613)
  arc A3264 (37.2277, 7.3905) -> (37.0032, 7.615) centre (37.1155, 7.5028) ccw
  line L1123 (35.2089, 8.1153) -> (34.56, 7.8465)
  arc A3265 (38.0059, 7.7045) -> (37.9562, 8.0181) centre (37.9811, 7.8613) ccw
  line L1124 (38.6801, 7.7506) -> (38.4539, 7.8241)
  arc A3266 (36.6722, 7.9588) -> (36.4477, 7.7343) centre (36.56, 7.8466) ccw
  line L1125 (38.8921, 7.6426) -> (38.6801, 7.7506)
  line L1126 (37.3079, 7.6426) -> (37.1155, 7.5028)
  arc A3267 (38.82, 7.5011) -> (38.9642, 7.784) centre (38.8921, 7.6425) ccw
  arc A3268 (39.2416, 7.0799) -> (39.4984, 7.2665) centre (39.37, 7.1732) ccw
  line L1127 (29.48, 15.0135) -> (30.1289, 14.7447)
  arc A3269 (24.2423, 15.1712) -> (24.0177, 15.3957) centre (24.13, 15.2835) ccw
  arc A3270 (31.5542, 7.6052) -> (31.7787, 7.3807) centre (31.6665, 7.493) ccw
  line L1128 (40.0599, 15.1094) -> (40.2861, 15.0359)
  arc A3271 (29.0007, 14.8668) -> (28.8792, 15.1601) centre (28.94, 15.0135) ccw
  line L1129 (39.8479, 15.2174) -> (40.0599, 15.1094)
  line L1130 (37.7489, 14.7447) -> (38.4511, 14.7447)
  arc A3272 (32.7296, 7.9686) -> (32.6081, 8.262) centre (32.6689, 8.1153) ccw
  arc A3273 (27.5889, 14.9034) -> (27.5889, 14.586) centre (27.5889, 14.7447) ccw
  line L1131 (24.003, 15.1565) -> (24.13, 15.2835)
  line L1132 (32.02, 7.8465) -> (31.6665, 7.493)
  arc A3274 (24.1153, 14.5557) -> (23.8907, 14.3312) centre (24.003, 14.4435) ccw
  line L1133 (30.9534, 7.493) -> (24.003, 14.4434)
  arc A3275 (25.7511, 14.586) -> (25.7511, 14.9034) centre (25.7511, 14.7447) ccw
  arc A3276 (33.4319, 8.262) -> (33.3104, 7.9686) centre (33.3712, 8.1153) ccw
  line L1134 (27.5889, 14.7447) -> (28.2911, 14.7447)
  arc A3277 (23.8442, 14.4434) -> (24.1617, 14.4434) centre (24.003, 14.4434) ccw
  arc A3278 (40.237, 14.8849) -> (40.3352, 15.1869) centre (40.2861, 15.0359) ccw
  arc A3279 (33.3711, 7.9565) -> (33.3711, 8.274) centre (33.3711, 8.1152) ccw
  arc A3280 (34.0807, 14.8668) -> (33.9592, 15.1601) centre (34.02, 15.0135) ccw
  arc A3281 (33.9077, 15.1257) -> (34.1322, 14.9012) centre (34.02, 15.0135) ccw
  arc A3282 (32.1323, 7.7343) -> (31.9078, 7.9588) centre (32.0201, 7.8466) ccw
  arc A3283 (34.6208, 15.1601) -> (34.4993, 14.8668) centre (34.5601, 15.0135) ccw
  line L1135 (34.02, 7.8465) -> (33.3711, 8.1153)
  line L1136 (34.02, 15.0135) -> (34.29, 15.2835)
  line L1137 (24.4, 15.0135) -> (25.0489, 14.7447)
  arc A3284 (26.8278, 14.9012) -> (27.0523, 15.1257) centre (26.9401, 15.0135) ccw
  arc A3285 (30.1289, 14.9034) -> (30.1289, 14.586) centre (30.1289, 14.7447) ccw
  arc A3286 (28.2911, 14.586) -> (28.2911, 14.9034) centre (28.2911, 14.7447) ccw
  arc A3287 (28.2304, 14.8914) -> (28.3519, 14.598) centre (28.2911, 14.7447) ccw
  arc A3288 (39.6619, 15.5753) -> (39.4373, 15.3508) centre (39.5496, 15.4631) ccw
  arc A3289 (34.4023, 15.3957) -> (34.1777, 15.1712) centre (34.29, 15.2834) ccw
  arc A3290 (26.4607, 14.8668) -> (26.3392, 15.1601) centre (26.4, 15.0134) ccw
  arc A3291 (26.7823, 15.3957) -> (26.5577, 15.1712) centre (26.67, 15.2835) ccw
  line L1138 (36.83, 15.2835) -> (37.1, 15.0135)
  arc A3292 (33.3104, 14.8914) -> (33.4319, 14.598) centre (33.3712, 14.7447) ccw
  line L1139 (36.56, 15.0135) -> (36.83, 15.2835)
  arc A3293 (31.3677, 15.1257) -> (31.5922, 14.9012) centre (31.4799, 15.0135) ccw
  arc A3294 (32.6689, 8.274) -> (32.6689, 7.9565) centre (32.6689, 8.1152) ccw
  arc A3295 (39.1607, 14.8668) -> (39.0392, 15.1601) centre (39.1, 15.0135) ccw
  arc A3296 (35.2089, 14.9034) -> (35.2089, 14.586) centre (35.2089, 14.7447) ccw
  arc A3297 (24.4608, 15.1601) -> (24.3393, 14.8668) centre (24.4001, 15.0135) ccw
  arc A3298 (27.0008, 15.1601) -> (26.8793, 14.8668) centre (26.9401, 15.0135) ccw
  arc A3299 (31.9593, 7.9932) -> (32.0808, 7.6999) centre (32.0201, 7.8466) ccw
  arc A3300 (27.5281, 14.598) -> (27.6496, 14.8914) centre (27.5889, 14.7447) ccw
  arc A3301 (30.8311, 14.586) -> (30.8311, 14.9034) centre (30.8311, 14.7447) ccw
  line L1140 (39.6555, 15.3572) -> (39.8479, 15.2174)
  arc A3302 (30.9534, 7.6517) -> (30.9534, 7.3342) centre (30.9534, 7.493) ccw
  line L1141 (24.003, 14.4434) -> (24.003, 15.1565)
  arc A3303 (39.9878, 14.968) -> (40.1319, 15.2509) centre (40.0599, 15.1094) ccw
  line L1142 (26.94, 15.0135) -> (27.5889, 14.7447)
  arc A3304 (36.9423, 15.1712) -> (36.7177, 15.3957) centre (36.83, 15.2835) ccw
  arc A3305 (37.7489, 14.9034) -> (37.7489, 14.586) centre (37.7489, 14.7447) ccw
  arc A3306 (39.92, 15.3589) -> (39.7758, 15.076) centre (39.8479, 15.2175) ccw
  arc A3307 (28.8277, 15.1257) -> (29.0522, 14.9012) centre (28.94, 15.0135) ccw
  arc A3308 (33.9592, 7.6999) -> (34.0807, 7.9932) centre (34.02, 7.8466) ccw
  arc A3309 (24.1617, 15.1565) -> (23.8442, 15.1565) centre (24.003, 15.1565) ccw
  line L1143 (26.67, 15.2835) -> (26.94, 15.0135)
  arc A3310 (30.8412, 7.3807) -> (31.0657, 7.6053) centre (30.9534, 7.493) ccw
  line L1144 (28.2911, 14.7447) -> (28.94, 15.0135)
  line L1145 (32.6689, 8.1153) -> (32.02, 7.8465)
  arc A3311 (39.7488, 15.4857) -> (39.5621, 15.2288) centre (39.6555, 15.3573) ccw
  line L1146 (33.3711, 8.1153) -> (32.6689, 8.1153)
  arc A3312 (24.2878, 14.9012) -> (24.5123, 15.1257) centre (24.4001, 15.0135) ccw
  arc A3313 (24.9881, 14.598) -> (25.1096, 14.8914) centre (25.0489, 14.7447) ccw
  line L1147 (31.75, 15.2835) -> (32.02, 15.0135)
  line L1148 (35.9111, 14.7447) -> (36.56, 15.0135)
  arc A3314 (30.7704, 14.8914) -> (30.8919, 14.598) centre (30.8312, 14.7447) ccw
  line L1149 (32.02, 15.0135) -> (32.6689, 14.7447)
  arc A3315 (36.9878, 14.9012) -> (37.2123, 15.1257) centre (37.1001, 15.0135) ccw
  arc A3316 (32.6689, 14.9034) -> (32.6689, 14.586) centre (32.6689, 14.7447) ccw
  arc A3317 (31.5407, 14.8668) -> (31.4192, 15.1601) centre (31.4799, 15.0135) ccw
  line L1150 (39.5496, 15.4631) -> (39.6555, 15.3572)
  line L1151 (34.56, 15.0135) -> (35.2089, 14.7447)
  arc A3318 (36.4477, 15.1257) -> (36.6722, 14.9012) centre (36.56, 15.0135) ccw
  line L1152 (33.3711, 14.7447) -> (34.02, 15.0135)
  arc A3319 (31.8623, 15.3957) -> (31.6377, 15.1712) centre (31.75, 15.2835) ccw
  line L1153 (40.2861, 15.0359) -> (40.5211, 14.9987)
  arc A3320 (36.9423, 15.3957) -> (36.7177, 15.1712) centre (36.83, 15.2834) ccw
  arc A3321 (35.9111, 14.586) -> (35.9111, 14.9034) centre (35.9111, 14.7447) ccw
  arc A3322 (32.6081, 14.598) -> (32.7296, 14.8914) centre (32.6689, 14.7447) ccw
  line L1154 (35.2089, 14.7447) -> (35.9111, 14.7447)
  line L1155 (31.48, 15.0135) -> (31.75, 15.2835)
  arc A3323 (32.0808, 15.1601) -> (31.9593, 14.8668) centre (32.0201, 15.0134) ccw
  line L1156 (39.1, 15.0135) -> (39.5496, 15.4631)
  arc A3324 (38.9877, 15.1257) -> (39.2122, 14.9012) centre (39.1, 15.0135) ccw
  arc A3325 (39.5432, 15.245) -> (39.7677, 15.4695) centre (39.6555, 15.3573) ccw
  arc A3326 (37.6881, 14.598) -> (37.8096, 14.8914) centre (37.7489, 14.7447) ccw
  arc A3327 (31.8623, 15.1712) -> (31.6377, 15.3957) centre (31.75, 15.2835) ccw
  arc A3328 (31.9078, 14.9012) -> (32.1323, 15.1257) centre (32.0201, 15.0135) ccw
  line L1157 (40.64, 14.9987) -> (40.64, 16.51)
  arc A3329 (41.8896, 15.9789) -> (42.1916, 15.8808) centre (42.0406, 15.9299) ccw
  arc A3330 (38.3904, 14.8914) -> (38.5119, 14.598) centre (38.4511, 14.7447) ccw
  arc A3331 (41.5123, 15.4695) -> (41.7368, 15.245) centre (41.6246, 15.3573) ccw
  arc A3332 (39.7546, 15.089) -> (39.9412, 15.3458) centre (39.8479, 15.2174) ccw
  arc A3333 (38.4511, 14.586) -> (38.4511, 14.9034) centre (38.4511, 14.7447) ccw
  arc A3334 (42.1513, 16.3513) -> (42.1513, 16.6688) centre (42.1513, 16.51) ccw
  line L1158 (30.8311, 14.7447) -> (31.48, 15.0135)
  arc A3335 (40.4962, 14.8419) -> (40.5459, 15.1555) centre (40.5211, 14.9987) ccw
  arc A3336 (40.5211, 15.1574) -> (40.5211, 14.84) centre (40.5211, 14.9987) ccw
  line L1159 (41.7928, 15.5255) -> (41.9326, 15.7179)
  arc A3337 (35.8504, 14.8914) -> (35.9719, 14.598) centre (35.9112, 14.7447) ccw
  line L1160 (42.1141, 16.1561) -> (42.1513, 16.3911)
  arc A3338 (42.31, 16.6289) -> (41.9925, 16.6289) centre (42.1513, 16.6289) ccw
  line L1161 (40.64, 16.51) -> (40.64, 14.9987)
  arc A3339 (39.6619, 15.3508) -> (39.4373, 15.5753) centre (39.5496, 15.4631) ccw
  line L1162 (42.1513, 16.51) -> (42.1513, 16.6289)
  line L1163 (34.29, 15.2835) -> (34.56, 15.0135)
  arc A3340 (33.3711, 14.586) -> (33.3711, 14.9034) centre (33.3711, 14.7447) ccw
  arc A3341 (36.6207, 14.8668) -> (36.4992, 15.1601) centre (36.56, 15.0134) ccw
  line L1164 (37.1, 15.0135) -> (37.7489, 14.7447)
  line L1165 (32.6689, 14.7447) -> (33.3711, 14.7447)
  arc A3342 (37.1608, 15.1601) -> (37.0393, 14.8668) centre (37.1, 15.0134) ccw
  arc A3343 (35.1481, 14.598) -> (35.2696, 14.8914) centre (35.2088, 14.7447) ccw
  arc A3344 (40.1089, 15.2604) -> (40.0108, 14.9584) centre (40.0599, 15.1094) ccw
  line L1166 (38.4511, 14.7447) -> (39.1, 15.0135)
  arc A3345 (34.4478, 14.9012) -> (34.6723, 15.1257) centre (34.5601, 15.0135) ccw
  arc A3346 (40.64, 16.6688) -> (40.64, 16.3513) centre (40.64, 16.51) ccw
  line L1167 (41.2201, 15.1094) -> (41.4321, 15.2174)
  arc A3347 (34.4023, 15.1712) -> (34.1777, 15.3957) centre (34.29, 15.2835) ccw
  arc A3348 (41.9925, 16.51) -> (42.31, 16.51) centre (42.1513, 16.51) ccw
  arc A3349 (40.7987, 16.51) -> (40.4812, 16.51) centre (40.6399, 16.51) ccw
  arc A3350 (41.2692, 14.9584) -> (41.1711, 15.2604) centre (41.2202, 15.1094) ccw
  arc A3351 (40.4813, 16.51) -> (40.7988, 16.51) centre (40.6401, 16.51) ccw
  line L1168 (41.4321, 15.2174) -> (41.6245, 15.3572)
  arc A3352 (40.64, 16.6688) -> (40.64, 16.3513) centre (40.64, 16.51) ccw
  arc A3353 (40.4812, 16.51) -> (40.7987, 16.51) centre (40.6399, 16.51) ccw
  arc A3354 (40.64, 17.8625) -> (40.64, 18.18) centre (40.64, 18.0212) ccw
  arc A3355 (41.9925, 16.3911) -> (42.31, 16.3911) centre (42.1513, 16.3911) ccw
  arc A3356 (40.4812, 14.9987) -> (40.7987, 14.9987) centre (40.6399, 14.9987) ccw
  line L1169 (41.6245, 15.3572) -> (41.7928, 15.5255)
  arc A3357 (41.3388, 15.3458) -> (41.5254, 15.089) centre (41.4321, 15.2174) ccw
  arc A3358 (41.6643, 15.6188) -> (41.9212, 15.4321) centre (41.7927, 15.5255) ccw
  line L1170 (42.0406, 15.9299) -> (42.1141, 16.1561)
  line L1171 (40.9939, 15.0359) -> (41.2201, 15.1094)
  line L1172 (42.0406, 17.0901) -> (41.9326, 17.3021)
  arc A3359 (40.64, 16.6687) -> (40.64, 16.3512) centre (40.64, 16.5099) ccw
  line L1173 (40.2861, 17.9841) -> (40.0599, 17.9106)
  arc A3360 (40.3352, 17.8331) -> (40.237, 18.1351) centre (40.2861, 17.9841) ccw
  arc A3361 (39.7758, 17.944) -> (39.92, 17.6611) centre (39.8479, 17.8026) ccw
  line L1174 (42.1513, 16.51) -> (40.64, 16.51)
  arc A3362 (40.64, 15.1575) -> (40.64, 14.84) centre (40.64, 14.9988) ccw
  arc A3363 (41.9631, 16.8148) -> (42.2651, 16.913) centre (42.1141, 16.8639) ccw
  arc A3364 (39.9412, 17.6741) -> (39.7546, 17.931) centre (39.8479, 17.8025) ccw
  arc A3365 (39.4373, 17.6692) -> (39.6619, 17.4446) centre (39.5496, 17.5569) ccw
  arc A3366 (42.3081, 16.3662) -> (41.9945, 16.4159) centre (42.1513, 16.3911) ccw
  arc A3367 (42.1916, 17.1392) -> (41.8896, 17.0411) centre (42.0406, 17.0902) ccw
  arc A3368 (41.0187, 14.8791) -> (40.9691, 15.1927) centre (40.9939, 15.0359) ccw
  line L1175 (39.1, 18.0065) -> (38.4511, 18.2753)
  line L1176 (41.9326, 15.7179) -> (42.0406, 15.9299)
  arc A3369 (40.1319, 17.7691) -> (39.9878, 18.052) centre (40.0599, 17.9106) ccw
  arc A3370 (41.8041, 17.2088) -> (42.061, 17.3954) centre (41.9326, 17.3021) ccw
  arc A3371 (40.9448, 15.1869) -> (41.043, 14.8849) centre (40.9939, 15.0359) ccw
  line L1177 (40.5211, 18.0213) -> (40.2861, 17.9841)
  arc A3372 (40.7341, 15.1555) -> (40.7838, 14.8419) centre (40.7589, 14.9987) ccw
  arc A3373 (41.905, 15.4132) -> (41.6805, 15.6377) centre (41.7928, 15.5254) ccw
  arc A3374 (40.7988, 16.51) -> (40.4813, 16.51) centre (40.6401, 16.51) ccw
  line L1178 (40.64, 14.9987) -> (40.7589, 14.9987)
  arc A3375 (41.5042, 15.076) -> (41.36, 15.3589) centre (41.4321, 15.2175) ccw
  arc A3376 (42.1513, 16.3512) -> (42.1513, 16.6687) centre (42.1513, 16.5099) ccw
  line L1179 (42.1141, 16.8639) -> (42.0406, 17.0901)
  arc A3377 (42.061, 15.6246) -> (41.8041, 15.8112) centre (41.9326, 15.7179) ccw
  line L1180 (40.64, 16.51) -> (42.1513, 16.51)
  arc A3378 (41.9573, 16.1809) -> (42.2709, 16.1313) centre (42.1141, 16.1561) ccw
  line L1181 (40.5211, 14.9987) -> (40.64, 14.9987)
  arc A3379 (42.2709, 16.8887) -> (41.9573, 16.8391) centre (42.1141, 16.8639) ccw
  arc A3380 (42.2651, 16.107) -> (41.9631, 16.2052) centre (42.1141, 16.1561) ccw
  arc A3381 (41.9945, 16.6041) -> (42.3081, 16.6538) centre (42.1513, 16.629) ccw
  arc A3382 (40.7589, 14.84) -> (40.7589, 15.1575) centre (40.7589, 14.9988) ccw
  arc A3383 (40.64, 16.3512) -> (40.64, 16.6687) centre (40.64, 16.5099) ccw
  arc A3384 (40.4813, 14.9987) -> (40.7988, 14.9987) centre (40.6401, 14.9987) ccw
  line L1182 (42.1513, 16.6289) -> (42.1141, 16.8639)
  line L1183 (40.7589, 14.9987) -> (40.9939, 15.0359)
  arc A3385 (41.7179, 15.2288) -> (41.5312, 15.4857) centre (41.6246, 15.3573) ccw
  arc A3386 (40.64, 16.6687) -> (40.64, 16.3512) centre (40.64, 16.5099) ccw
  arc A3387 (40.3109, 15.1927) -> (40.2613, 14.8791) centre (40.2861, 15.0359) ccw
  arc A3388 (42.182, 15.8578) -> (41.8991, 16.0019) centre (42.0406, 15.9299) ccw
  arc A3389 (42.31, 16.51) -> (41.9925, 16.51) centre (42.1513, 16.51) ccw
  arc A3390 (40.7988, 16.51) -> (40.4813, 16.51) centre (40.6401, 16.51) ccw
  arc A3391 (40.64, 14.8399) -> (40.64, 15.1574) centre (40.64, 14.9986) ccw
  line L1184 (42.1513, 16.3911) -> (42.1513, 16.51)
  arc A3392 (41.1481, 15.2509) -> (41.2922, 14.968) centre (41.2202, 15.1094) ccw
  arc A3393 (41.7911, 15.79) -> (42.074, 15.6458) centre (41.9325, 15.7179) ccw
  arc A3394 (38.4511, 18.1165) -> (38.4511, 18.434) centre (38.4511, 18.2752) ccw
  arc A3395 (40.7838, 18.1781) -> (40.7341, 17.8645) centre (40.7589, 18.0213) ccw
  arc A3396 (37.2123, 17.8943) -> (36.9878, 18.1188) centre (37.1001, 18.0066) ccw
  line L1185 (39.6555, 17.6628) -> (39.5496, 17.5569)
  line L1186 (40.7589, 18.0213) -> (40.64, 18.0213)
  arc A3397 (37.7489, 18.434) -> (37.7489, 18.1165) centre (37.7489, 18.2752) ccw
  line L1187 (41.7928, 17.4945) -> (41.6245, 17.6628)
  arc A3398 (41.6805, 17.3823) -> (41.905, 17.6068) centre (41.7928, 17.4945) ccw
  arc A3399 (41.7368, 17.775) -> (41.5123, 17.5505) centre (41.6246, 17.6627) ccw
  line L1188 (40.64, 18.0213) -> (40.64, 16.51)
  line L1189 (26.94, 18.0065) -> (26.67, 17.7365)
  arc A3400 (26.5577, 17.8488) -> (26.7823, 17.6243) centre (26.67, 17.7366) ccw
  arc A3401 (39.4373, 17.4446) -> (39.6619, 17.6692) centre (39.5496, 17.5569) ccw
  arc A3402 (41.8991, 17.0181) -> (42.182, 17.1622) centre (42.0406, 17.0902) ccw
  line L1190 (29.21, 17.7365) -> (28.94, 18.0065)
  arc A3403 (41.5312, 17.5343) -> (41.7179, 17.7912) centre (41.6246, 17.6628) ccw
  arc A3404 (34.1777, 17.8488) -> (34.4023, 17.6243) centre (34.29, 17.7366) ccw
  arc A3405 (34.6723, 17.8943) -> (34.4478, 18.1188) centre (34.5601, 18.0066) ccw
  arc A3406 (27.6496, 18.1286) -> (27.5281, 18.422) centre (27.5889, 18.2753) ccw
  arc A3407 (40.5211, 18.18) -> (40.5211, 17.8625) centre (40.5211, 18.0212) ccw
  arc A3408 (40.0108, 18.0616) -> (40.1089, 17.7596) centre (40.0599, 17.9106) ccw
  arc A3409 (41.5254, 17.931) -> (41.3388, 17.6741) centre (41.4321, 17.8026) ccw
  arc A3410 (41.2922, 18.052) -> (41.1481, 17.7691) centre (41.2202, 17.9106) ccw
  arc A3411 (39.0392, 17.8599) -> (39.1607, 18.1532) centre (39.1, 18.0065) ccw
  arc A3412 (37.0393, 18.1532) -> (37.1608, 17.8599) centre (37.1, 18.0065) ccw
  arc A3413 (40.7589, 17.8625) -> (40.7589, 18.18) centre (40.7589, 18.0212) ccw
  arc A3414 (40.7987, 18.0213) -> (40.4812, 18.0213) centre (40.6399, 18.0213) ccw
  line L1191 (41.4321, 17.8026) -> (41.2201, 17.9106)
  arc A3415 (39.2122, 18.1188) -> (38.9877, 17.8943) centre (39.1, 18.0065) ccw
  line L1192 (41.9326, 17.3021) -> (41.7928, 17.4945)
  line L1193 (31.75, 17.7365) -> (31.48, 18.0065)
  line L1194 (39.5496, 17.5569) -> (39.1, 18.0065)
  arc A3416 (41.36, 17.6611) -> (41.5042, 17.944) centre (41.4321, 17.8026) ccw
  arc A3417 (41.1711, 17.7596) -> (41.2692, 18.0616) centre (41.2202, 17.9106) ccw
  arc A3418 (32.6689, 18.434) -> (32.6689, 18.1165) centre (32.6689, 18.2752) ccw
  line L1195 (37.1, 18.0065) -> (36.83, 17.7365)
  line L1196 (41.6245, 17.6628) -> (41.4321, 17.8026)
  arc A3419 (37.8096, 18.1286) -> (37.6881, 18.422) centre (37.7489, 18.2753) ccw
  line L1197 (41.2201, 17.9106) -> (40.9939, 17.9841)
  line L1198 (40.0599, 17.9106) -> (39.8479, 17.8026)
  line L1199 (40.64, 18.0213) -> (40.5211, 18.0213)
  arc A3420 (40.4813, 16.51) -> (40.7988, 16.51) centre (40.6401, 16.51) ccw
  line L1200 (40.64, 16.51) -> (40.64, 18.0213)
  arc A3421 (42.074, 17.3742) -> (41.7911, 17.23) centre (41.9325, 17.3021) ccw
  arc A3422 (39.5621, 17.7912) -> (39.7488, 17.5343) centre (39.6555, 17.6627) ccw